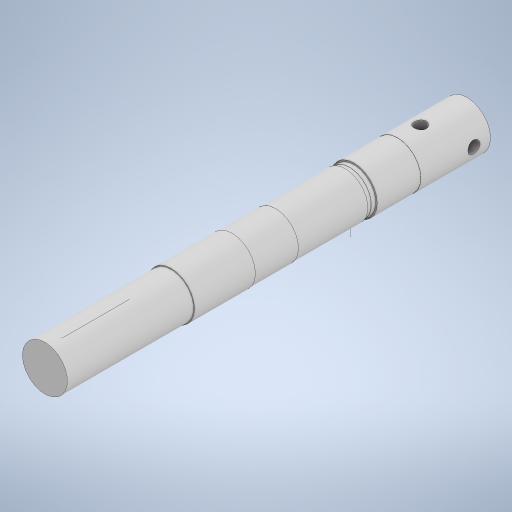
# Autodesk Inventor part: Mangon_Conduccion
Saved by Autodesk Inventor 2024 (Build 280153000, 153)
## iProperties
Created: 2026-01-05
Part Number: Mangon_Conduccion
Material: Generic
Document SubType Name: Modeling
Designer: eduso
Density: 1 g/cm^3
Appearance: Default
Testero_007: 5,000 mm
Espacio_008: 50,000 mm
Inteerior_Tubo_009: 80,000 mm
Author: eduso
Autodesk Inventor part; units mm, degrees
ref_plane "YZ Plane" through (0, 0, 0) normal (1, 0, 0) x (0, 1, 0)
ref_plane "XY Plane" through (0, 0, 0) normal (0, 0, 1) x (1, 0, 0)
sketch "Sketch1" plane through (0, 0, 0) normal (0, 1, 0) x (-1, 0, 0)
  line L0 (24.85, 6) -> (26.05, 6)
  line L1 (26.05, 6) -> (26.05, 86)
  line L2 (26.05, 86) -> (26.35, 86)
  line L3 (26.35, 86) -> (26.35, 136)
  line L4 (26.35, 136) -> (26.85, 136)
  line L5 (26.85, 136) -> (26.85, 206)
  line L6 (26.85, 206) -> (25.85, 206)
  line L7 (25.85, 206) -> (25.85, 246)
  line L8 (25.85, 246) -> (25.85, 246)
  line L9 (25.85, 246) -> (25.85, 351)
  line L10 (25.85, 351) -> (0, 351)
  line L11 (0, 189.8856) -> (0, -122.7414) construction
  line L12 (24.85, 6) -> (24.85, 1)
  line L13 (0, 351) -> (0, 0)
  line L14 (24.85, 1) -> (25.05, 1)
  line L15 (25.05, 1) -> (25.05, -4)
  line L16 (25.05, -4) -> (26.75, -4)
  line L17 (26.75, -4) -> (26.75, -54)
  line L18 (26.75, -54) -> (26.95, -54)
  line L19 (26.95, -54) -> (26.95, -134)
  line L20 (26.95, -134) -> (0, -134)
  line L21 (0, 0) -> (0, -134)
  line L22 (24.85, 1) -> (25.05, 1)
  dimension "d0" = 105
  dimension "d3" = 70
  dimension "d2" = 80
  dimension "d4" = 5
  dimension "d15" = 40
  dimension "d16" = 50
  dimension "d69" = 25.85
  dimension "d70" = 26.85
  dimension "d71" = 26.05
  dimension "d78" = 24.85
  dimension "d82" = 5
  dimension "d83" = 50
  dimension "d84" = 25.05
  dimension "d85" = 26.95
  dimension "d86" = 80
  dimension "d87" = 25.85
  dimension "d88" = 26.35
  dimension "d89" = 26.75
  constraints: 46 end point, 10 perpendicular, 3 horizontal, 3 vertical, 2 collinear, 1 point on line, 3 other
  measures "d0" distance of L8.end L9.end
  measures "d3" distance of L4.end L5.end
  measures "d2" distance of L0.end L1.end
  measures "d4" distance of L0.start L12.end
  measures "d15" distance of L6.end L7.end
  measures "d16" distance of L2.end L3.end
  measures "d69" distance between parallel lines of L13 L9
  measures "d70" distance between parallel lines of L13 L5
  measures "d71" distance between parallel lines of L1 L13
  measures "d78" distance between parallel lines of L11 L12
  measures "d82" distance of L14.end L15.end
  measures "d83" distance of L16.end L17.end
  measures "d84" distance between parallel lines of L11 L15
  measures "d85" distance between parallel lines of L21 L19
  measures "d86" distance of L18.end L19.end
  measures "d87" distance between parallel lines of L13 L7
  measures "d88" distance between parallel lines of L11 L3
  measures "d89" distance between parallel lines of L11 L17
ref_plane "Work Plane1" through (0, 15, 0) normal (0, 1, 0) x (-1, 0, 0)
sketch "Sketch2" plane through (0, 15, 0) normal (0, 1, 0) x (-1, 0, 0)
  arc A0 (-5, 260) -> (5, 260) centre (0, 260) ccw
  arc A1 (5, 335) -> (-5, 335) centre (0, 335) ccw
  line L0 (-5, 335) -> (-5, 260)
  line L1 (5, 335) -> (5, 260)
  line L2 (0, 0) -> (0, 401.4271) construction
  dimension "d18" = 10
  dimension "d19" = 10
  dimension "d65" = 260
  dimension "d68" = 75
  constraints: 6 end point, 4 point on circle, 3 tangent, 2 centre point, 2 point on line, 1 parallel, 1 vertical
  measures "d18" diameter of A0
  measures "d19" diameter of A1
  measures "d65" distance of L2.start A0.centre
  measures "d68" distance of A1.centre A0.centre
sketch "Sketch3" plane through (0, 15, 0) normal (0, 1, 0) x (-1, 0, 0)
  circle A0 centre (0, -80) radius 7
  point P0 (0, 0)
  dimension "d22" = 14
  dimension "d66" = 80
  constraints: 1 centre point
  measures "d22" diameter of A0
  measures "d66" distance of point (0, 0) A0.centre
sketch "Sketch4" plane through (0, 0, 0) normal (1, 0, 0) x (0, 1, 0)
  circle A0 centre (0, -115) radius 7
  point P0 (0, 0)
  dimension "d28" = 14
  dimension "d67" = 115
  constraints: 1 centre point
  measures "d28" diameter of A0
  measures "d67" distance of point (0, 0) A0.centre
revolve "Revolution1" add sketch "Sketch1" angle 360 about axis through (0, 0, 351) along (0, 0, -1)
extrude "Extrusion4" cut sketch "Sketch2" along normal blind 10
extrude "Extrusion5" cut sketch "Sketch3" along normal blind 20 and the other way blind 45
extrude "Extrusion6" cut sketch "Sketch4" along normal blind 35 and the other way blind 30
sketch "Sketch5" plane through (0, 0, 0) normal (0, 1, 0) x (-1, 0, 0)
  line L0 (24.85, 6) -> (24.85, 1) projected
  point P0 (0, 0)
sketch "Sketch6" plane through (0, 0, 0) normal (1, 0, 0) x (0, 1, 0)
  line L0 (0, 0) -> (-46.2751, 0) construction
  constraints: 2 end point, 1 horizontal
equation "\"espesor_testero\" = 5"
equation "\"espesor_brida\" = 5"
body "Solid4"
